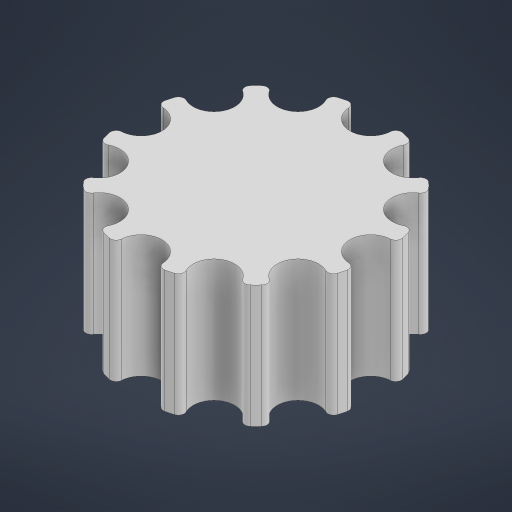
# Autodesk Inventor part: 5mm_HTD_Pully
Saved by Autodesk Inventor 2024.2 (Build 282272000, 272)
## iProperties
Created: 2026-01-08
Part Number: 5mm_HTD_Pully
Material: Generic
Document SubType Name: Modeling
Designer: 4aida
Density: 1 g/cm^3
Appearance: Default
Author: 4aida
Autodesk Inventor part; units mm, degrees
ref_plane "YZ Plane" through (0, 0, 0) normal (1, 0, 0) x (0, 1, 0)
ref_plane "XZ Plane" through (0, 0, 0) normal (0, 1, 0) x (-1, 0, 0)
ref_plane "XY Plane" through (0, 0, 0) normal (0, 0, 1) x (1, 0, 0)
sketch "Sketch2" plane through (0, 0, 0) normal (0, 1, 0) x (-1, 0, 0)
  circle A0 centre (0, 0) radius 8.9778 construction
  circle A1 centre (0, 0) radius 6.9178 construction
  arc A2 (0, -6.9178) -> (-1.5221, -8.3486) centre (0, -8.4428) ccw
  line L0 (0, 0) -> (0, -8.9778) construction
  line L1 (0, 0) -> (-2.3236, -8.6719) construction
  arc A3 (-2.0494, -8.7407) -> (-1.5221, -8.3486) centre (-1.9513, -8.3221) ccw
  arc A4 (-2.8562, -7.9912) -> (-3.4589, -5.991) centre (-4.2214, -7.3117) ccw
  arc A5 (-2.8562, -7.9912) -> (-2.5955, -8.5944) centre (-2.4712, -8.1828) ccw
  arc A6 (-2.5955, -8.5944) -> (-2.0494, -8.7407) centre (0, 0) ccw
  arc A7 (2.5955, -8.5944) -> (2.8562, -7.9912) centre (2.4712, -8.1828) ccw
  arc A8 (1.5221, -8.3486) -> (0, -6.9178) centre (0, -8.4428) ccw
  arc A9 (1.5221, -8.3486) -> (2.0494, -8.7407) centre (1.9513, -8.3221) ccw
  arc A10 (2.0494, -8.7407) -> (2.5955, -8.5944) centre (0, 0) ccw
  arc A11 (3.4589, -5.991) -> (2.8562, -7.9912) centre (4.2214, -7.3117) ccw
  arc A12 (6.545, -6.1452) -> (6.4691, -5.4925) centre (6.2315, -5.8509) ccw
  arc A13 (5.4925, -6.4691) -> (3.4589, -5.991) centre (4.2214, -7.3117) ccw
  arc A14 (5.4925, -6.4691) -> (6.1452, -6.545) centre (5.8509, -6.2315) ccw
  arc A15 (6.1452, -6.545) -> (6.545, -6.1452) centre (0, 0) ccw
  arc A16 (5.991, -3.4589) -> (6.4691, -5.4925) centre (7.3117, -4.2214) ccw
  arc A17 (8.7407, -2.0494) -> (8.3486, -1.5221) centre (8.3221, -1.9513) ccw
  arc A18 (7.9912, -2.8562) -> (5.991, -3.4589) centre (7.3117, -4.2214) ccw
  arc A19 (7.9912, -2.8562) -> (8.5944, -2.5955) centre (8.1828, -2.4712) ccw
  arc A20 (8.5944, -2.5955) -> (8.7407, -2.0494) centre (0, 0) ccw
  arc A21 (6.9178, 0) -> (8.3486, -1.5221) centre (8.4428, 0) ccw
  arc A22 (8.5944, 2.5955) -> (7.9912, 2.8562) centre (8.1828, 2.4712) ccw
  arc A23 (8.3486, 1.5221) -> (6.9178, 0) centre (8.4428, 0) ccw
  arc A24 (8.3486, 1.5221) -> (8.7407, 2.0494) centre (8.3221, 1.9513) ccw
  arc A25 (8.7407, 2.0494) -> (8.5944, 2.5955) centre (0, 0) ccw
  arc A26 (5.991, 3.4589) -> (7.9912, 2.8562) centre (7.3117, 4.2214) ccw
  arc A27 (6.1452, 6.545) -> (5.4925, 6.4691) centre (5.8509, 6.2315) ccw
  arc A28 (6.4691, 5.4925) -> (5.991, 3.4589) centre (7.3117, 4.2214) ccw
  arc A29 (6.4691, 5.4925) -> (6.545, 6.1452) centre (6.2315, 5.8509) ccw
  arc A30 (6.545, 6.1452) -> (6.1452, 6.545) centre (0, 0) ccw
  arc A31 (3.4589, 5.991) -> (5.4925, 6.4691) centre (4.2214, 7.3117) ccw
  arc A32 (2.0494, 8.7407) -> (1.5221, 8.3486) centre (1.9513, 8.3221) ccw
  arc A33 (2.8562, 7.9912) -> (3.4589, 5.991) centre (4.2214, 7.3117) ccw
  arc A34 (2.8562, 7.9912) -> (2.5955, 8.5944) centre (2.4712, 8.1828) ccw
  arc A35 (2.5955, 8.5944) -> (2.0494, 8.7407) centre (0, 0) ccw
  arc A36 (0, 6.9178) -> (1.5221, 8.3486) centre (0, 8.4428) ccw
  arc A37 (-2.5955, 8.5944) -> (-2.8562, 7.9912) centre (-2.4712, 8.1828) ccw
  arc A38 (-1.5221, 8.3486) -> (0, 6.9178) centre (0, 8.4428) ccw
  arc A39 (-1.5221, 8.3486) -> (-2.0494, 8.7407) centre (-1.9513, 8.3221) ccw
  arc A40 (-2.0494, 8.7407) -> (-2.5955, 8.5944) centre (0, 0) ccw
  arc A41 (-3.4589, 5.991) -> (-2.8562, 7.9912) centre (-4.2214, 7.3117) ccw
  arc A42 (-6.545, 6.1452) -> (-6.4691, 5.4925) centre (-6.2315, 5.8509) ccw
  arc A43 (-5.4925, 6.4691) -> (-3.4589, 5.991) centre (-4.2214, 7.3117) ccw
  arc A44 (-5.4925, 6.4691) -> (-6.1452, 6.545) centre (-5.8509, 6.2315) ccw
  arc A45 (-6.1452, 6.545) -> (-6.545, 6.1452) centre (0, 0) ccw
  arc A46 (-5.991, 3.4589) -> (-6.4691, 5.4925) centre (-7.3117, 4.2214) ccw
  arc A47 (-8.7407, 2.0494) -> (-8.3486, 1.5221) centre (-8.3221, 1.9513) ccw
  arc A48 (-7.9912, 2.8562) -> (-5.991, 3.4589) centre (-7.3117, 4.2214) ccw
  arc A49 (-7.9912, 2.8562) -> (-8.5944, 2.5955) centre (-8.1828, 2.4712) ccw
  arc A50 (-8.5944, 2.5955) -> (-8.7407, 2.0494) centre (0, 0) ccw
  arc A51 (-6.9178, 0) -> (-8.3486, 1.5221) centre (-8.4428, 0) ccw
  arc A52 (-8.5944, -2.5955) -> (-7.9912, -2.8562) centre (-8.1828, -2.4712) ccw
  arc A53 (-8.3486, -1.5221) -> (-6.9178, 0) centre (-8.4428, 0) ccw
  arc A54 (-8.3486, -1.5221) -> (-8.7407, -2.0494) centre (-8.3221, -1.9513) ccw
  arc A55 (-8.7407, -2.0494) -> (-8.5944, -2.5955) centre (0, 0) ccw
  arc A56 (-5.991, -3.4589) -> (-7.9912, -2.8562) centre (-7.3117, -4.2214) ccw
  arc A57 (-6.1452, -6.545) -> (-5.4925, -6.4691) centre (-5.8509, -6.2315) ccw
  arc A58 (-6.4691, -5.4925) -> (-5.991, -3.4589) centre (-7.3117, -4.2214) ccw
  arc A59 (-6.4691, -5.4925) -> (-6.545, -6.1452) centre (-6.2315, -5.8509) ccw
  arc A60 (-6.545, -6.1452) -> (-6.1452, -6.545) centre (0, 0) ccw
  arc A61 (-3.4589, -5.991) -> (-5.4925, -6.4691) centre (-4.2214, -7.3117) ccw
  point P0 (2.3236, -8.6719)
  point P1 (6.3483, -6.3483)
  point P2 (8.6719, -2.3236)
  point P3 (8.6719, 2.3236)
  point P4 (6.3483, 6.3483)
  point P5 (2.3236, 8.6719)
  point P6 (-2.3236, 8.6719)
  point P7 (-6.3483, 6.3483)
  point P8 (-8.6719, 2.3236)
  point P9 (3.4589, -5.991)
  point P10 (6.9178, 0)
  point P11 (5.991, 3.4589)
  point P12 (3.4589, 5.991)
  point P13 (0, 6.9178)
  point P14 (-5.991, 3.4589)
  point P15 (-3.1307, -4.309)
  point P16 (0, -6.9178)
  point P17 (-8.6719, -2.3236)
  point P18 (-6.3483, -6.3483)
  dimension "d1" = 13.8356
  dimension "d2" = 17.9556
  dimension "d3" = 15
  dimension "d4" = 3.05
  dimension "d5" = 0.86
  dimension "d8" = 360
  constraints: 135 point on circle, 62 centre point, 5 symmetric about line, 4 end point, 3 tangent, 2 coincident, 2 point on line, 1 vertical, 207 other
  measures "d1" diameter of A1
  measures "d2" diameter of A0
  measures "d3" angle of L1 L0
  measures "d4" diameter of A2
  measures "d5" diameter of A3
extrude "Extrusion1" add sketch "Sketch2" along normal blind 9
body "Solid1"
